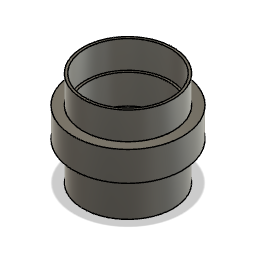
Federkörper v8 (Autodesk Fusion 360 design; units mm, degrees)
Autodesk Fusion 360 part; units mm, degrees
sketch "Sketch1" plane through (0, 0, 0) normal (0, 0, 1) x (1, 0, 0)
  line L0 (45, 44.5) -> (45, -55.5)
  line L1 (45, -55.5) -> (47.5, -55.5)
  line L2 (47.5, -55.5) -> (47.5, -15.5)
  line L3 (47.5, -15.5) -> (57.5, -15.5)
  line L4 (57.5, -15.5) -> (57.5, 15.5)
  line L5 (57.5, 15.5) -> (47.5, 15.5)
  line L6 (47.5, 15.5) -> (47.5, 44.5)
  line L7 (47.5, 44.5) -> (45, 44.5)
  line L8 (0, 0) -> (57.5, 0) construction
  line L9 (45, 15.5) -> (42.5, 15.5)
  line L10 (42.5, 15.5) -> (42.5, -15.5)
  line L11 (42.5, -15.5) -> (45, -15.5)
  dimension "d1" = 45
  dimension "d2" = 47.5
  dimension "d4" = 31
  dimension "d8" = 29
  dimension "d9" = 40
  dimension "d10" = 100
  dimension "d11" = 57.5
  dimension "d12" = 42.5
  constraint vertical L0
  constraint perpendicular L0 L1
  constraint perpendicular L1 L2
  constraint perpendicular L0 L3
  constraint perpendicular L3 L4
  constraint perpendicular L0 L5
  constraint perpendicular L5 L6
  constraint perpendicular L0 L7
  constraint coincident L8.start origin
  constraint coincident L4 L8.end
  constraint perpendicular L4 L8
  constraint collinear L2 L6
  constraint midpoint L4 L8.end
  constraint coincident L0 L9.start
  constraint perpendicular L0 L9
  constraint perpendicular L9 L10
  constraint coincident L0 L11.end
  constraint perpendicular L0 L11
  constraint collinear L5 L9
  constraint collinear L3 L11
  measures "d1" distance of L8.start L0
  measures "d2" distance of L8.start L2
  measures "d4" distance of L3.end L4.end
  measures "d8" distance of L5 L7
  measures "d9" distance of L1 L3
  measures "d10" distance of L1 L7
  measures "d11" distance of L8.start L8.end
  measures "d12" distance of L8.start L10
revolve "Revolve1" add sketch "Sketch1" angle 360 about axis through (0, 1.75, 0) along (0, 1, 0)
equation "d1 = ( 90 / 2 ) * 1 mm"
equation "d2 = ( 95 / 2 ) * 1 mm"
equation "d11 = ( 115 / 2 ) * 1 mm"
equation "d12 = ( 85 / 2 ) * 1 mm"
